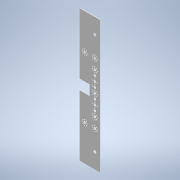
# Autodesk Inventor part: plate1
Saved by Autodesk Inventor 2020.1 (Build 241239000, 239)
## iProperties
Created: 2019-12-06
Part Number: plate1
Material: Generic
Document SubType Name: Modeling
Designer: tbloo
Density: 1 g/cm^3
Appearance: Default
Author: tbloo
Autodesk Inventor part; units mm, degrees
ref_plane "YZ Plane" through (0, 0, 0) normal (1, 0, 0) x (0, 1, 0)
ref_plane "XZ Plane" through (0, 0, 0) normal (0, 1, 0) x (-1, 0, 0)
ref_plane "XY Plane" through (0, 0, 0) normal (0, 0, 1) x (1, 0, 0)
sketch "Sketch1" plane through (0, 0, 0) normal (0, 0, 1) x (1, 0, 0)
  circle A0 centre (32, -32) radius 4.7 projected
  circle A1 centre (32, -352) radius 4.7 projected
  line L0 (48, -210) -> (48, -398) projected
  arc A2 (46, -400) -> (48, -398) centre (46, -398) ccw projected
  line L1 (46, -400) -> (-14, -400) projected
  line L2 (-16, -398) -> (-16, -210) projected
  arc A3 (-16, -398) -> (-14, -400) centre (-14, -398) ccw projected
  arc A4 (-14, -208) -> (-16, -210) centre (-14, -210) ccw projected
  line L3 (48, -114.5) -> (48, -269.5) projected
  line L4 (48, 14) -> (48, -174) projected
  arc A5 (-16, -174) -> (-14, -176) centre (-14, -174) ccw projected
  line L5 (-16, -174) -> (-16, 14) projected
  line L6 (-14, 16) -> (46, 16) projected
  arc A6 (-14, 16) -> (-16, 14) centre (-14, 14) ccw projected
  arc A7 (48, 14) -> (46, 16) centre (46, 14) ccw projected
  circle A8 centre (32, -120) radius 1.85 projected
  circle A9 centre (37.6569, -122.3431) radius 1.85 projected
  circle A10 centre (40, -128) radius 1.85 projected
  circle A11 centre (37.6569, -133.6569) radius 1.85 projected
  circle A12 centre (32, -136) radius 1.85 projected
  circle A13 centre (32, -128) radius 4 projected
  circle A14 centre (26.3431, -133.6569) radius 1.85 projected
  circle A15 centre (23.8856, -128.1676) radius 1.85 projected
  circle A16 centre (26.3431, -122.3431) radius 1.85 projected
  circle A17 centre (32, -144) radius 4 projected
  circle A18 centre (32, -152) radius 1.85 projected
  circle A19 centre (32, -160) radius 4 projected
  circle A20 centre (40, -160) radius 1.85 projected
  circle A21 centre (24, -160) radius 1.85 projected
  circle A22 centre (32, -168) radius 1.85 projected
  circle A23 centre (32, -176) radius 4 projected
  circle A24 centre (23.8856, -176.1676) radius 1.85 projected
  circle A25 centre (32, -184) radius 1.85 projected
  circle A26 centre (37.6569, -186.3431) radius 1.85 projected
  circle A27 centre (40, -192) radius 1.85 projected
  circle A28 centre (32, -192) radius 4 projected
  circle A29 centre (37.6569, -197.6569) radius 1.85 projected
  circle A30 centre (24, -192) radius 1.85 projected
  circle A31 centre (26.3431, -186.3431) radius 1.85 projected
  circle A32 centre (26.3431, -197.6569) radius 1.85 projected
  circle A33 centre (32, -200) radius 1.85 projected
  circle A34 centre (32, -208) radius 4 projected
  circle A35 centre (32, -216) radius 1.85 projected
  circle A36 centre (40, -224) radius 1.85 projected
  circle A37 centre (32, -232) radius 1.85 projected
  circle A38 centre (24, -224) radius 1.85 projected
  circle A39 centre (32, -224) radius 4 projected
  circle A40 centre (32, -240) radius 4 projected
  circle A41 centre (32, -248) radius 1.85 projected
  circle A42 centre (37.6569, -250.3431) radius 1.85 projected
  circle A43 centre (40, -256) radius 1.85 projected
  circle A44 centre (37.6569, -261.6569) radius 1.85 projected
  circle A45 centre (32, -264) radius 1.85 projected
  circle A46 centre (26.3431, -261.6569) radius 1.85 projected
  circle A47 centre (24, -256) radius 1.85 projected
  circle A48 centre (26.3431, -250.3431) radius 1.85 projected
  circle A49 centre (32, -256) radius 4 projected
  circle A50 centre (37.6569, -101.6569) radius 1.85 projected
  circle A51 centre (40, -96) radius 1.85 projected
  circle A52 centre (37.6569, -90.3431) radius 1.85 projected
  circle A53 centre (32, -88) radius 1.85 projected
  circle A54 centre (32, -96) radius 4 projected
  circle A55 centre (26.3431, -90.3431) radius 1.85 projected
  circle A56 centre (24, -96) radius 1.85 projected
  circle A57 centre (26.3431, -101.6569) radius 1.85 projected
  circle A58 centre (32, -104) radius 1.85 projected
  circle A59 centre (24, -288.0038) radius 1.85 projected
  circle A60 centre (26.3431, -293.6606) radius 1.85 projected
  circle A61 centre (32, -296.0038) radius 1.85 projected
  circle A62 centre (37.6569, -293.6606) radius 1.85 projected
  circle A63 centre (40, -288.0038) radius 1.85 projected
  circle A64 centre (37.6569, -282.3469) radius 1.85 projected
  circle A65 centre (32, -280.0038) radius 1.85 projected
  circle A66 centre (26.3431, -282.3469) radius 1.85 projected
  circle A67 centre (32, -288.0038) radius 4 projected
  line L7 (-14, -176) -> (16, -176)
  line L8 (16, -176) -> (16, -208)
  line L9 (16, -208) -> (-14, -208)
  circle A68 centre (0, -288) radius 4 projected
  circle A69 centre (5.6569, -293.6569) radius 1.85 projected
  circle A70 centre (8, -288) radius 1.85 projected
  circle A71 centre (5.6569, -282.3431) radius 1.85 projected
  circle A72 centre (0, -280) radius 1.85 projected
  circle A73 centre (-5.6569, -282.3431) radius 1.85 projected
  circle A74 centre (-8, -288) radius 1.85 projected
  circle A75 centre (-5.6569, -293.6569) radius 1.85 projected
  circle A76 centre (0, -296) radius 1.85 projected
  circle A77 centre (5.6569, -90.3431) radius 1.85 projected
  circle A78 centre (8, -96) radius 1.85 projected
  circle A79 centre (5.6569, -101.6569) radius 1.85 projected
  circle A80 centre (0, -104) radius 1.85 projected
  circle A81 centre (-5.6569, -101.6569) radius 1.85 projected
  circle A82 centre (-8, -96) radius 1.85 projected
  circle A83 centre (-5.6569, -90.3431) radius 1.85 projected
  circle A84 centre (0, -88) radius 1.85 projected
  circle A85 centre (0, -96) radius 4 projected
  point P0 (0, 0)
  constraints: 6 end point, 2 perpendicular, 1 horizontal
extrude "Extrusion1" add sketch "Sketch1" along normal blind 2
body "Solid1"
